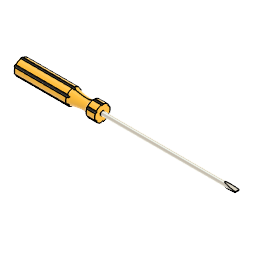
PS70DrillScrewdriverAssemblyFusionFile (Autodesk Fusion 360 archive; units mm, degrees)
design "PS70 ScrewDriver"
part number: 2025-09-18-19-45-50-265
Autodesk Fusion 360 part; units mm, degrees
sketch "Sketch1" plane through (0, 0, 0) normal (0, 1, 0) x (1, 0, 0)
  line L0 (-167.35, 0) -> (132.65, 0)
  line L1 (-89.6, 0) -> (0, 0)
  line L2 (0, 0) -> (0, -8.6286)
  line L3 (0, -8.6286) -> (-89.6, -8.6286)
  line L4 (-89.6, -8.6286) -> (-89.6, 0)
  line L5 (0, -2.3) -> (150.4, -2.3)
  line L6 (150.4, -2.3) -> (150.4, 0)
  line L7 (150.4, 0) -> (0, 0)
  line L8 (0, 0) -> (0, -2.3)
  spline S0 degree 5 poles (-32.3672, -8.6286) (-32.2548, -8.5496) (-32.0088, -8.3926) (-31.5762, -8.1601) (-30.8721, -7.856) (-29.7791, -7.4865) (-28.4781, -7.13) (-26.9828, -6.7908) (-25.3199, -6.4761) (-23.5353, -6.1966) (-21.6902, -5.966) (-19.8536, -5.7987) (-18.0951, -5.7083) (-16.4783, -5.7057) (-15.0531, -5.7973) (-13.8498, -5.9831) (-12.8682, -6.2539) (-12.0785, -6.5915) (-11.4365, -6.9745) (-10.8948, -7.3816) (-10.4165, -7.7972) (-10.0704, -8.1305) (-9.8284, -8.3798) (-9.6748, -8.5457) (-9.6, -8.6286) knots 0 0 0 0 0 0 0.05 0.1 0.15 0.2 0.25 0.3 0.35 0.4 0.45 0.5 0.55 0.6 0.65 0.7 0.75 0.8 0.85 0.9 0.95 1 1 1 1 1 1
  ellipse E0 centre (-89.6, 0) end of major axis (-89.6, -8.6286) minor radius 3.7 (-93.3, 0) -> (-85.9, 0) ccw
  point P0 (-26.3948, -6.6873)
  point P1 (-14.3646, -5.9194)
  point P2 (-11.0371, -7.2846)
  dimension "d1" = 300
  dimension "d2" = 89.6
  dimension "d3" = 8.6286
  dimension "d4" = 150.4
  dimension "d5" = 2.3
  dimension "d8" = 9.6
  dimension "d9" = 7.4
  constraint horizontal L0
  constraint coincident L1.end L0
  constraint horizontal L1
  constraint vertical L2
  constraint horizontal L3
  constraint vertical L4
  constraint coincident L1.end L2.start
  constraint horizontal L5
  constraint vertical L6
  constraint horizontal L7
  constraint vertical L8
  constraint collinear L2 L8
  constraint collinear L0 L7
  constraint coincident L3 S0.start
  constraint coincident L3 S0.end
  constraint coincident L1.start L4.end
  measures "d1" distance of L0.start L0.end
  measures "d2" distance of L2.end L3.end
  measures "d3" distance of L1.start L3.end
  measures "d4" distance of L6.end L1.end
  measures "d5" distance of L5.end L6.end
  measures "d8" distance of L2.end S0.end
revolve "Revolve1" add sketch "Sketch1" angle 360 about axis through (-167.35, 0, 0) along (1, 0, 0) contours L0 L4 E0 | L0 L1 L4 E0 | L0 L1 L2 L3 L8 S0 E0 | L0 L2 L5 L6 L7 L8
sketch "Sketch2" plane through (0, 0, 0) normal (0, 1, 0) x (1, 0, 0)
  line L0 (170, 0) -> (-110, 0)
  line L1 (150.4, -0.37) -> (136.4, -2.3)
  line L2 (150.4, 0.37) -> (136.4, 2.3)
  line L3 (136.4, -2.3) -> (150.4, -2.3)
  line L4 (150.4, -2.3) -> (150.4, -0.37)
  line L5 (150.4011, 2.3) -> (136.4, 2.3)
  line L6 (150.4, 2.3) -> (150.4, -2.3)
  dimension "d10" = 136.4
  dimension "d11" = 2.3
  dimension "d12" = 150.4
  dimension "d13" = 0.37
  dimension "d14" = 90
  dimension "d15" = 90
  constraint horizontal L0
  constraint coincident origin L0
  constraint symmetric L0 L1.start L2.start
  constraint symmetric L0 L1.end L2.end
  constraint horizontal L3
  measures "d10" horizontal distance of origin L1.end
  measures "d11" distance of L0 L1.end
  measures "d12" horizontal distance of origin L1.start
  measures "d13" distance of L0 L1.start
  measures "d14" angle of L3 L4
  measures "d15" angle of L5 L6
extrude "Extrude1" cut sketch "Sketch2" along normal mid plane 40
sketch "Sketch3" plane through (0, 0, 0) normal (1, 0, 0) x (0, 1, 0)
  circle A0 centre (0, 0) radius 8.75
  circle A1 centre (0, 8.75) radius 1.1913
  line L0 (0, 0) -> (0, 8.6286)
  circle A2 centre (-7.5777, 4.375) radius 1.1913
  circle A3 centre (-7.5777, -4.375) radius 1.1913
  circle A4 centre (0, -8.75) radius 1.1913
  circle A5 centre (7.5777, -4.375) radius 1.1913
  circle A6 centre (7.5777, 4.375) radius 1.1913
  dimension "d19" = 360
  dimension "d22" = 17.5
  constraint coincident A0.centre L0.start
  constraint coincident A0 A1.centre
  constraint coincident A1.centre L0
  measures "d22" diameter of A0
extrude "Extrude2" cut sketch "Sketch3" along normal mid plane 600 contours A0 A6 | A0 A6 | A0 A5 | A0 A1 | A0 A1 | A0 A4 | A0 A2 | A0 A3 picked at (7.2153, -4.1985) picked at (0.0284, -8.3479) picked at (-7.2401, 4.1547) picked at (-7.2401, -4.1547)
equation "d2 = 93.3 mm - 3.7 mm"
equation "d3 = ( 60.4 * ( 2 / 7 ) ) / 2 * 1 mm"
equation "d10 = 150.4 mm - 14 mm"

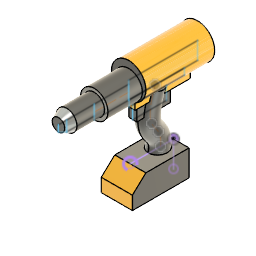
design "PS70 Drill"
part number: 2025-09-18-18-29-46-875
Autodesk Fusion 360 part; units mm, degrees
sketch "Sketch2" plane through (0, 0, 0) normal (1, 0, 0) x (0, 1, 0)
  line L0 (0, 0) -> (-113.2, 0)
  line L1 (-113.2, 0) -> (-113.2, 26.7)
  line L2 (-86.3, 51.9) -> (0, 51.9)
  line L3 (0, 51.9) -> (0, 0)
  line L4 (-86.3, 51.9) -> (-113.2, 26.7)
  dimension "d1" = 113.2
  dimension "d2" = 51.9
  dimension "d3" = 86.3
  dimension "d4" = 26.7
  constraint horizontal L0
  constraint vertical L1
  constraint horizontal L2
  constraint vertical L3
  constraint coincident L0.start L3.end
  measures "d1" distance of L0.start L0.end
  measures "d2" distance of L0.start L2.end
  measures "d3" distance of L2.end L2.start
  measures "d4" distance of L0.end L1.end
extrude "Extrude1" add sketch "Sketch2" along normal blind 62.2 makes body 1
ref_plane "WorkPlane1" through (31.1, 0, 0) normal (1, 0, 0) x (0, 1, 0)
sketch "Sketch3" plane through (31.1, 0, 0) normal (1, 0, 0) x (0, 1, 0)
  line L0 (47.8879, 197.95) -> (-89.5121, 197.95)
  line L1 (-89.5121, 197.95) -> (-89.5121, 163.6)
  line L2 (-89.5121, 163.6) -> (47.8879, 163.6)
  line L3 (47.8879, 163.6) -> (47.8879, 197.95)
  line L4 (0, 51.9) -> (0, 0)
  line L5 (-86.3, 51.9) -> (0, 51.9)
  line L6 (-89.5121, 191) -> (-158.2121, 191)
  line L7 (-158.2121, 191) -> (-158.2121, 163.6)
  line L8 (-158.2121, 163.6) -> (-89.5121, 163.6)
  line L9 (-89.5121, 163.6) -> (-89.5121, 191)
  line L10 (-89.5121, 177.3) -> (-158.2121, 177.3) construction
  line L11 (-158.2121, 191) -> (-213.1721, 191)
  line L12 (-213.1721, 191) -> (-213.1721, 170.45)
  line L13 (-213.1721, 170.45) -> (-158.2121, 170.45)
  line L14 (-158.2121, 170.45) -> (-158.2121, 191)
  line L15 (-213.1721, 170.45) -> (-213.1721, 191)
  line L16 (-213.1721, 191) -> (-229.6121, 191)
  line L17 (-229.6121, 191) -> (-229.6121, 178.3)
  line L18 (-229.6121, 178.3) -> (-213.1721, 170.45)
  spline S0 degree 5 poles (-26.0256, 51.9) (-25.8292, 53.4797) (-25.5289, 56.5687) (-25.3557, 60.9909) (-25.6831, 66.462) (-27.0217, 72.5971) (-29.2397, 78.079) (-32.2063, 83.0319) (-35.6533, 87.7033) (-39.2005, 92.4405) (-42.4377, 97.6159) (-44.9819, 103.5758) (-46.5608, 110.5628) (-47.0265, 118.7038) (-46.3099, 128.0539) (-44.3968, 138.6184) (-41.9207, 148.0265) (-39.5419, 155.6097) (-37.7257, 160.8978) (-36.7601, 163.6) knots 0 0 0 0 0 0 0.066667 0.133333 0.2 0.266667 0.333333 0.4 0.466667 0.533333 0.6 0.666667 0.733333 0.8 0.866667 0.933333 1 1 1 1 1 1 construction
  line L19 (21.6823, 163.6) -> (-88.6177, 163.6)
  line L20 (-88.6177, 163.6) -> (-88.6177, 151.3)
  line L21 (-88.6177, 151.3) -> (21.6823, 151.3)
  line L22 (21.6823, 151.3) -> (21.6823, 163.6)
  line L23 (-14.1079, 151.3) -> (-81.2298, 151.3)
  line L24 (-81.2298, 151.3) -> (-81.2298, 125.6)
  line L25 (-81.2298, 125.6) -> (-14.1079, 125.6)
  line L26 (-14.1079, 125.6) -> (-14.1079, 151.3)
  point P0 (-30.5104, 80)
  point P1 (-43.5557, 100.5876)
  dimension "d8" = 111.7
  dimension "d9" = 34.35
  dimension "d10" = 137.4
  dimension "d11" = 68.7
  dimension "d12" = 27.4
  dimension "d13" = 20.55
  dimension "d14" = 54.96
  dimension "d15" = 20.55
  dimension "d16" = 12.7
  dimension "d17" = 16.44
  dimension "d18" = 110.3
  dimension "d19" = 12.3
  dimension "d20" = 25.7
  constraint horizontal L0
  constraint vertical L1
  constraint horizontal L2
  constraint vertical L3
  constraint horizontal L6
  constraint vertical L7
  constraint horizontal L8
  constraint vertical L9
  constraint coincident L1.end L9
  constraint collinear L2 L8
  constraint midpoint L9 L10.start
  constraint midpoint L7 L10.end
  constraint horizontal L11
  constraint vertical L12
  constraint horizontal L13
  constraint vertical L14
  constraint coincident L10.end L14
  constraint collinear L6 L11
  constraint vertical L15
  constraint perpendicular L15 L16
  constraint perpendicular L16 L17
  constraint coincident L11.end L12.start
  constraint coincident L5 S0.start
  constraint coincident L2 S0.end
  constraint horizontal L19
  constraint vertical L20
  constraint horizontal L21
  constraint vertical L22
  constraint collinear L2 L19
  constraint horizontal L23
  constraint vertical L24
  constraint horizontal L25
  constraint vertical L26
  constraint collinear L21 L23
  measures "d8" distance of L2 L5
  measures "d9" distance of L0.start L2.end
  measures "d10" distance of L0.start L0.end
  measures "d11" distance of L7.end L1.end
  measures "d12" distance of L6.end L7.end
  measures "d13" distance of L11.end L12.end
  measures "d14" distance of L12.end L13.end
  measures "d15" distance of L12.end L11.end
  measures "d16" distance of L16.end L17.end
  measures "d17" distance of L11.end L16.end
  measures "d18" distance of L20.end L21.end
  measures "d19" distance of L19.start L21.end
  measures "d20" distance of L23.end L24.end
revolve "Revolve1" add sketch "Sketch3" angle 360 about axis through (31.1, -89.5121, 191) along (0, -1, 0) separate body contours L1 L6 L7 L8 L9 L14 | L7 L11 L12 L13 L14 L15 | L12 L15 L16 L17 L18 makes body 2
revolve "Revolve2" add sketch "Sketch3" angle 360 about axis through (31.1, 47.8879, 197.95) along (0, -1, 0) contours L0 L1 L2 L3 L9 L19 bodies 2
extrude "Extrude2" add sketch "Sketch3" along normal mid plane 23.4 separate body contours L2 L19 L20 L21 L22 L23 makes body 3
extrude "Extrude3" add sketch "Sketch3" along normal mid plane 15.9 contours L21 L23 L24 L25 L26 bodies 3
sketch "Sketch5" plane through (0, 0, 51.9) normal (0, 0, 1) x (-1, 0, 0)
  line L0 (0, 0) -> (0, 86.3)
  line L1 (0, 86.3) -> (-62.2, 86.3)
  line L2 (-62.2, 86.3) -> (-62.2, 0)
  line L3 (-62.2, 0) -> (0, 0)
  ellipse E0 centre (-30, 30) end of major axis (-48.66, 30) minor radius 19.45
  line L4 (-11.34, 30) -> (-48.66, 30) construction
  line L5 (-30, 49.45) -> (-30, 10.55) construction
  dimension "d27" = 38.9
  dimension "d28" = 37.32
  constraint coincident E0 L4.start
  constraint coincident E0 L4.end
  constraint coincident E0 L5.start
  constraint coincident E0 L5.end
  constraint horizontal L4
  measures "d28" distance of E0
sweep "Sweep1" add profiles "Sketch5" path "Sketch3" along S0 section 1 contours E0 bodies 1 2 3
equation "d9 = ( 68.7 / 2 ) * 1 mm"
equation "d10 = ( 2 * 68.7 ) * 1 mm"
equation "d12 = ( 54.8 / 2 ) * 1 mm"
equation "d13 = ( 41.1 / 2 ) * 1 mm"
equation "d14 = ( ( 4 / 5 ) * 68.7 ) * 1 mm"
equation "d15 = ( 41.1 / 2 ) * 1 mm"
equation "d16 = ( 25.4 / 2 ) * 1 mm"
equation "d17 = ( 41.1 * ( 2 / 5 ) ) * 1 mm"
equation "d23 = ( 23.4 / 2 ) * 1 mm"
equation "d25 = ( 15.9 / 2 ) * 1 mm"
equation "d28 = ( ( 3 / 5 ) * 62.2 ) * 1 mm"
